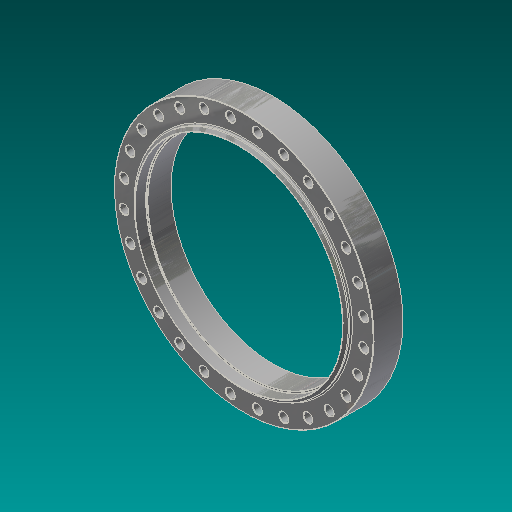
# Autodesk Inventor part: A1-19027-300-03 Alco flange - 30in CL150
Saved by Autodesk Inventor 2017.3 (Build 213257000, 257)
## iProperties
Created: 2019-06-24
Part Number: A1-19027-300-03 Alco flange - 30in CL150
Material: Steel, Mild
Document SubType Name: Modeling
Designer: Graeme_Van_Dongen
Density: 7.85 g/cm^3
Appearance: Steel
Mass: 230260 g
Surface Area: 15470.2 cm^2
Volume: 29332.4 cm^3
Description: 30" CLASS 150 FF ALCO FLANGE, A350 LF2, Ø30 1/2" BORE, MATES TO 30" CLASS 150 B16.47 Ser.A
Author: Graeme_Van_Dongen
Autodesk Inventor part; units mm, degrees
ref_plane "YZ Plane" through (0, 0, 0) normal (1, 0, 0) x (0, 1, 0)
ref_plane "XZ Plane" through (0, 0, 0) normal (0, 1, 0) x (-1, 0, 0)
ref_plane "XY Plane" through (0, 0, 0) normal (0, 0, 1) x (1, 0, 0)
sketch "Sketch1" plane through (0, 0, 0) normal (1, 0, 0) x (0, 1, 0)
  line L0 (0, 0) -> (0, 130.175)
  line L1 (428.625, 0) -> (393.7, 0)
  line L2 (393.7, 0) -> (393.7, 130.175)
  line L3 (393.7, 130.175) -> (395.2875, 130.175)
  line L4 (395.2875, 130.175) -> (406.4, 121.6481)
  line L5 (406.4, 121.6481) -> (406.4, 116.205)
  arc A0 (406.4, 116.205) -> (411.48, 111.125) centre (411.48, 116.205) ccw
  line L6 (411.48, 111.125) -> (492.125, 111.125)
  line L7 (492.125, 111.125) -> (492.125, 1.5875)
  line L8 (492.125, 1.5875) -> (428.625, 1.5875) construction
  line L9 (428.625, 1.5875) -> (428.625, 0) construction
  line L10 (428.625, 0) -> (492.125, 0)
  line L11 (492.125, 0) -> (492.125, 1.5875)
  point P0 (406.4, 111.125)
  dimension "d0" = 130.175
  dimension "d1" = 984.25
  dimension "d2" = 111.125
  dimension "d3" = 857.25
  dimension "d4" = 1.5875
  dimension "d5" = 812.8
  dimension "d6" = 787.4
  dimension "d7" = 812.8
  dimension "d8" = 37.5
  dimension "d9" = 11.1125
  dimension "d10" = 5.08
  constraints: 24 end point, 6 perpendicular, 4 point on line, 2 horizontal, 2 point on circle, 2 tangent, 1 centre point, 1 parallel, 1 vertical
  measures "d0" distance of L0.start L0.end
  measures "d1" diameter of L7 L0
  measures "d2" distance between parallel lines of L6 L1
  measures "d3" diameter of L9 L0
  measures "d4" distance between parallel lines of L8 L1
  measures "d5" diameter of L4.end L0
  measures "d6" diameter of L2 L0
  measures "d7" diameter of point (406.4, 111.125) L0
  measures "d8" angle of L3 L4
  measures "d9" horizontal distance of L3.end L4.end
  measures "d10" radius of A0
revolve "Revolution1" add sketch "Sketch1" angle 360 about axis through (0, 0, 0) along (0, 0, 1)
sketch "Sketch2" plane through (0, 0, 111.125) normal (0, 0, 1) x (1, 0, 0)
  line L0 (0, -688.975) -> (0, 688.975) construction
  line L1 (-51.1902, -454.3252) -> (51.1902, 454.3252) construction
  point P0 (0, 0)
  dimension "d12" = 914.4
  dimension "d13" = 6.429
  constraints: 2 end point, 1 coincident, 1 midpoint
  measures "d12" distance of L1.start L1.end
  measures "d13" angle of L0 L1
hole "Hole1" at (51.1902, 454.3252, 111.125) direction (0, 0, -1) diameter 34.925 end through all
chamfer "Chamfer1" distance 1.5875 angle 45 2 edges at (51.1902, 471.7877, 111.125) (51.1902, 471.7877, 0)
pattern_circular "Circular Pattern1" count 28 over 360 about axis through (0, 0, -10) along (0, 0, 1) of "Hole1", "Chamfer1"
chamfer "Chamfer2" distance 1.5875 angle 45 1 edges at (0, -492.125, 111.125)
sketch "Sketch3" plane through (0, 0, 0) normal (0, 0, -1) x (-1, 0, 0)
  circle A0 centre (0, 0) radius 393.7 projected
  circle A1 centre (0, 0) radius 387.35
  dimension "d30" = 774.7
  constraints: 1 centre point, 1 coincident
  measures "d30" diameter of A1
extrude "Extrusion1" add sketch "Sketch3" against normal blind 88.9
fillet "Fillet1" radius 0.7937 1 edges at (0, -393.7, 88.9)
chamfer "Chamfer3" distance 0.7937 angle 45 1 edges at (387.35, 0, 88.9)
equation "\"d0\" = Length"
equation "\"d1\" = OutsideDiameter"
equation "\"d2\" = Thickness"
equation "\"d3\" = RFDiameter"
equation "\"d4\" = RFThickness"
equation "\"d5\" = CasingDiameter"
equation "\"d6\" = Bore"
equation "\"d7\" = HubDiameter"
equation "\"d8\" = WeldBevelAngle"
equation "\"d9\" = WeldBevelSize"
equation "\"d10\" = HubRadius"
equation "\"d12\" = BCD"
equation "\"d14\" = HoleDiameter"
equation "\"d21\" = HoleChamfer"
equation "\"d27\" = RimChamfer"
equation "\"OutsideDiameter\" = 984.25"
equation "\"Thickness\" = 111.125"
equation "\"Length\" = 130.175"
equation "\"RFDiameter\" = 857.25"
equation "\"CasingDiameter\" = 812.8"
equation "\"Bore\" = 787.4"
equation "\"HoleDiameter\" = 34.925"
equation "\"BCD\" = 914.4"
equation "\"RFThickness\" = 1.5875"
equation "\"WeldBevelAngle\" = 37.5deg"
equation "\"HubDiameter\" = CasingDiameter"
equation "\"HoleChamfer\" = 1.5875"
equation "\"RimChamfer\" = 1.5875"
equation "\"HubRadius\" = 5.08"
equation "\"WeldBevelSize\" = 11.1125"
body "Solid1"
